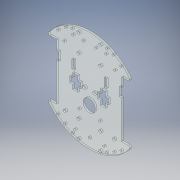
# Autodesk Inventor part: Part2_Estructura pequeña
Saved by Autodesk Inventor 2019 (Build 230136000, 136)
## iProperties
Created: 2023-05-02
Part Number: Part2_Estructura pequeña
Material: Generic
Document SubType Name: Modeling
Designer: Tecneu Technology
Density: 1 g/cm^3
Appearance: Glazing
Author: Tecneu Technology
Autodesk Inventor part; units mm, degrees
ref_plane "YZ Plane" through (0, 0, 0) normal (1, 0, 0) x (0, 1, 0)
ref_plane "XZ Plane" through (0, 0, 0) normal (0, 1, 0) x (-1, 0, 0)
ref_plane "XY Plane" through (0, 0, 0) normal (0, 0, 1) x (1, 0, 0)
sketch "Sketch1" plane through (0, 0, 0) normal (0, 0, 1) x (1, 0, 0)
  ellipse E0 centre (-7.26, 0) end of major axis (-10.02, 0) minor radius 1.8
  ellipse E1 centre (7.26, 0) end of major axis (10.02, 0) minor radius 1.8
  line L0 (11.52, 0) -> (11.52, 3.95)
  line L1 (11.52, 3.95) -> (15.52, 3.95)
  line L2 (15.52, 3.95) -> (15.52, 9.95)
  line L3 (15.52, 9.95) -> (22.84, 9.95)
  line L4 (22.84, 9.95) -> (22.84, 3.95)
  line L5 (22.84, 3.95) -> (26.84, 3.95)
  line L6 (26.84, 3.95) -> (26.84, 0)
  line L7 (11.52, 0) -> (11.52, -3.95)
  line L8 (11.52, -3.95) -> (15.52, -3.95)
  line L9 (15.52, -3.95) -> (15.52, -9.95)
  line L10 (15.52, -9.95) -> (22.84, -9.95)
  line L11 (22.84, -9.95) -> (22.84, -3.95)
  line L12 (22.84, -3.95) -> (26.84, -3.95)
  line L13 (26.84, -3.95) -> (26.84, 0)
  line L14 (-11.52, 0) -> (-11.52, 3.95)
  line L15 (-11.52, 3.95) -> (-15.52, 3.95)
  line L16 (-15.52, 3.95) -> (-15.52, 9.95)
  line L17 (-15.52, 9.95) -> (-22.84, 9.95)
  line L18 (-22.84, 9.95) -> (-22.84, 3.95)
  line L19 (-22.84, 3.95) -> (-26.84, 3.95)
  line L20 (-26.84, 3.95) -> (-26.84, 0)
  line L21 (-11.52, 0) -> (-11.52, -3.95)
  line L22 (-11.52, -3.95) -> (-15.52, -3.95)
  line L23 (-15.52, -3.95) -> (-15.52, -9.95)
  line L24 (-15.52, -9.95) -> (-22.84, -9.95)
  line L25 (-22.84, -9.95) -> (-22.84, -3.95)
  line L26 (-22.84, -3.95) -> (-26.84, -3.95)
  line L27 (-26.84, -3.95) -> (-26.84, 0)
  circle A0 centre (0, -18) radius 8.5
  circle A1 centre (14.5, -29.5) radius 1.5
  circle A2 centre (-14.5, -29.5) radius 1.5
  circle A3 centre (15, -41.5) radius 2
  circle A4 centre (34, -41.5) radius 2
  circle A5 centre (-15, -41.5) radius 2
  circle A6 centre (-34, -41.5) radius 2
  circle A7 centre (-15, -65.5) radius 2
  circle A8 centre (15, -65.5) radius 2
  circle A9 centre (44, -50.5) radius 1.5
  circle A10 centre (-44, -50.5) radius 1.5
  circle A11 centre (0, -57) radius 1.5
  circle A12 centre (20, -57) radius 1.5
  circle A13 centre (34, -57) radius 1.5
  circle A14 centre (-20, -57) radius 1.5
  circle A15 centre (-34, -57) radius 1.5
  circle A16 centre (23.5, -63) radius 1.5
  circle A17 centre (-23.5, -63) radius 1.5
  line L28 (23.84, 13.95) -> (20.76, 13.95)
  line L29 (20.76, 13.95) -> (20.76, 25.98)
  line L30 (20.76, 25.98) -> (23.84, 25.98)
  line L31 (23.84, 25.98) -> (23.84, 13.95)
  line L32 (-23.84, 13.95) -> (-20.76, 13.95)
  line L33 (-20.76, 13.95) -> (-20.76, 25.98)
  line L34 (-20.76, 25.98) -> (-23.84, 25.98)
  line L35 (-23.84, 25.98) -> (-23.84, 13.95)
  circle A18 centre (15, 37) radius 2
  circle A19 centre (15, 62) radius 2
  circle A20 centre (-15, 37) radius 2
  circle A21 centre (-15, 62) radius 2
  circle A22 centre (35, 41.5) radius 1.5
  circle A23 centre (43.5, 50.5) radius 1.5
  circle A24 centre (-35, 41.5) radius 1.5
  circle A25 centre (-43.5, 50.5) radius 1.5
  circle A26 centre (8.5, 55) radius 1.5
  circle A27 centre (23, 55) radius 1.5
  circle A28 centre (-8.5, 55) radius 1.5
  circle A29 centre (-23, 55) radius 1.5
  circle A30 centre (33, 59) radius 1.5
  circle A31 centre (-33, 59) radius 1.5
  circle A32 centre (24, 62) radius 1.5
  circle A33 centre (-24, 62) radius 1.5
  line L36 (-45, 0) -> (-45, 13.95)
  line L37 (-45, 13.95) -> (-41.92, 13.95)
  line L38 (-41.92, 13.95) -> (-41.92, 25.98)
  line L39 (-41.92, 25.98) -> (-45, 25.98)
  line L40 (-45, 25.98) -> (-45, 38.75)
  line L41 (-45, 38.75) -> (-54.4375, 38.75)
  line L42 (-45, 0) -> (-45, -38.75)
  line L43 (-45, -38.75) -> (-54.4375, -38.75)
  line L44 (45, 0) -> (45, 13.95)
  line L45 (45, 13.95) -> (41.92, 13.95)
  line L46 (41.92, 13.95) -> (41.92, 25.98)
  line L47 (41.92, 25.98) -> (45, 25.98)
  line L48 (45, 25.98) -> (45, 38.75)
  line L49 (45, 38.75) -> (54.4375, 38.75)
  line L50 (45, 0) -> (45, -38.75)
  line L51 (45, -38.75) -> (54.4375, -38.75)
  arc A34 (-56.0386, -41.9485) -> (56.0386, -41.9485) centre (0, 0) ccw
  arc A35 (56.0386, 41.9485) -> (-56.0386, 41.9485) centre (0, 0) ccw
  arc A36 (-56.0386, 41.9485) -> (-54.4375, 38.75) centre (-54.4375, 40.75) ccw
  arc A37 (54.4375, 38.75) -> (56.0386, 41.9485) centre (54.4375, 40.75) ccw
  arc A38 (56.0386, -41.9485) -> (54.4375, -38.75) centre (54.4375, -40.75) ccw
  arc A39 (-54.4375, -38.75) -> (-56.0386, -41.9485) centre (-54.4375, -40.75) ccw
  point P0 (-58.2961, 38.75)
  point P1 (-58.2961, -38.75)
  point P2 (58.2961, 38.75)
  point P3 (58.2961, -38.75)
  dimension "d148" = 2
  constraints: 104 end point, 40 centre point, 16 point on circle, 12 perpendicular, 8 tangent, 4 point on line, 4 vertical, 3 equal radius, 2 coincident, 2 horizontal, 4 other
  measures "d148" radius of A36
extrude "Extrusion1" add sketch "Sketch1" along normal blind 2.4
body "Solid1"
